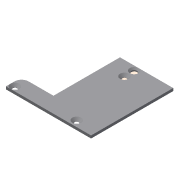
# Autodesk Inventor part: 11_Smartphone_Platform
Saved by Autodesk Inventor 2016 (Build 200138000, 138)
## iProperties
Created: 2017-01-03
Part Number: 11_Smartphone_Platform
Material: Generisch
Document SubType Name: Modeling
Designer: diederichbenedict
Density: 1 g/cm^3
Appearance: Vorgabe
Author: diederichbenedict
Autodesk Inventor part; units mm, degrees
ref_plane "YZ Plane" through (0, 0, 0) normal (1, 0, 0) x (0, 1, 0)
ref_plane "XZ Plane" through (0, 0, 0) normal (0, 1, 0) x (-1, 0, 0)
ref_plane "XY Plane" through (0, 0, 0) normal (0, 0, 1) x (1, 0, 0)
ref_plane "Arbeitsebene1" through (0, 0, 0) normal (0, 0, 1) x (1, 0, 0)
sketch "Skizze1" plane through (0, 0, 0) normal (0, 0, 1) x (1, 0, 0)
  circle A0 centre (-34, -41.2095) radius 2.25 projected
  line L0 (-29.75, -46.3143) -> (-39, -46.3143) projected
  line L1 (-29.75, -28.7171) -> (-29.75, -46.3143) projected
  line L2 (-31, -28.7171) -> (-29.75, -28.7171) projected
  arc A1 (-31, -28.7171) -> (-39, -36.7171) centre (-31, -36.7171) ccw projected
  line L3 (-39, -46.3143) -> (-39, -36.7171) projected
  line L4 (22, 46.3143) -> (22, 27.3143) projected
  line L5 (14, 46.3143) -> (22, 46.3143) projected
  line L6 (14, 27.3143) -> (14, 46.3143) projected
  line L7 (22, 27.3143) -> (14, 27.3143) projected
  circle A2 centre (18, 30.3143) radius 2.25 projected
  circle A3 centre (18, 41.3143) radius 3.2 projected
  line L8 (39, -36.6857) -> (39, -43.7095) projected
  arc A4 (39, -36.6857) -> (31, -28.6857) centre (31, -36.6857) ccw projected
  line L9 (30, -28.6857) -> (31, -28.6857) projected
  arc A5 (22, -20.6857) -> (30, -28.6857) centre (30, -20.6857) ccw projected
  line L10 (22, -18.1808) -> (22, -20.6857) projected
  line L11 (20, -18.1808) -> (22, -18.1808) projected
  line L12 (20, -43.7095) -> (20, -18.1808) projected
  line L13 (39, -43.7095) -> (20, -43.7095) projected
  circle A6 centre (34, -39.4595) radius 2.25 projected
  circle A7 centre (34, -58.6857) radius 4.25 construction
  circle A8 centre (-34, -58.6857) radius 4.25 construction
  circle A9 centre (18, 41.3143) radius 3.2 construction
  circle A10 centre (34, -39.4595) radius 2.25 construction
  circle A11 centre (-34, -41.2095) radius 2.25 construction
  circle A12 centre (18, 30.3143) radius 2.25 construction
  circle A13 centre (18, -14.7167) radius 2 construction
  circle A14 centre (18, 8.8143) radius 2 construction
  circle A15 centre (3.8024, -65.6857) radius 18.5 construction
  circle A16 centre (3, -8.6688) radius 3.05 construction
  arc A17 (-31, -28.7171) -> (-39, -36.7171) centre (-31, -36.7171) ccw construction
  line L14 (-11, -28.7171) -> (-31, -28.7171) construction
  arc A18 (-11, -28.7171) -> (-3, -20.7171) centre (-11, -20.7171) ccw construction
  line L15 (-3, 17.3143) -> (-3, -20.7171) construction
  arc A19 (5, 25.3143) -> (-3, 17.3143) centre (5, 17.3143) ccw construction
  line L16 (14, 25.3143) -> (5, 25.3143) construction
  line L17 (14, 46.3143) -> (14, 25.3143) construction
  line L18 (22, 46.3143) -> (14, 46.3143) construction
  line L19 (22, -20.6857) -> (22, 46.3143) construction
  arc A20 (22, -20.6857) -> (30, -28.6857) centre (30, -20.6857) ccw construction
  line L20 (31, -28.6857) -> (30, -28.6857) construction
  arc A21 (39, -36.6857) -> (31, -28.6857) centre (31, -36.6857) ccw construction
  line L21 (39, -79.0756) -> (39, -36.6857) construction
  arc A22 (31, -87.0756) -> (39, -79.0756) centre (31, -79.0756) ccw construction
  line L22 (-31, -87.0756) -> (31, -87.0756) construction
  arc A23 (-39, -79.0756) -> (-31, -87.0756) centre (-31, -79.0756) ccw construction
  line L23 (-39, -36.7171) -> (-39, -79.0756) construction
  circle A24 centre (3, 16.3312) radius 4 projected
  circle A25 centre (3, -33.6688) radius 4 projected
  circle A26 centre (3, 16.3312) radius 7.6 projected
  circle A27 centre (3, 16.3312) radius 4 projected
  circle A28 centre (3, 16.3312) radius 6 projected
  circle A29 centre (3, 16.3312) radius 6 projected
  line L24 (-39, -46.3143) -> (39, -46.3143)
  line L25 (39, -46.3143) -> (39, -43.7095)
  line L26 (-29.75, -28.7171) -> (-3, -28.7171)
  line L27 (-3, -28.7171) -> (-3, 46.3143)
  line L28 (-3, 46.3143) -> (22, 46.3143)
  line L29 (22, 46.3143) -> (22, -18.1808)
  line L30 (22, 46.3143) -> (57, 46.3143)
  line L31 (57, 46.3143) -> (57, -37.6857)
  line L32 (57, -37.6857) -> (22, -37.6857)
  line L33 (22, -37.6857) -> (22, 46.3143)
  line L34 (39, -46.3143) -> (57, -46.3143)
  line L35 (57, -46.3143) -> (57, -37.6857)
  line L36 (57, -37.6857) -> (39, -37.6857)
  line L37 (39, -37.6857) -> (39, -46.3143)
  point P0 (0, 0)
  dimension "d10" = 84
  dimension "d11" = 60
  constraints: 28 end point, 4 horizontal, 4 parallel, 3 perpendicular, 2 collinear, 2 point on line
  measures "d10" distance of L30.end L31.end
  measures "d11" distance between parallel lines of L31 L27
extrude "Extrusion1" add sketch "Skizze1" along normal blind 3 contours L0 L3 A1 L2 L1 | L1 L26 L27 A26 L28 L6 L7 L29 L11 L12 L13 L25 L24 | L25 L8 L32 L35 L34 | L13 L12 L11 L10 L33 L32 A6 L8 | A28 | L27 A26 | L32 A6 L33 A5 L9 A4 L8 | L8 A4 L9 A5 L10 L29 L4 L30 L31 L32 | L32 A6 | L4 L7 L6 L5 | A24 | A25 picked at (9.931, 15.2305) picked at (34.3207, -37.599)
sketch "Skizze2" plane through (0, 0, 0) normal (0, 0, -1) x (-1, 0, 0)
  circle A0 centre (-3, 16.3312) radius 4 projected
  circle A1 centre (-3, -33.6688) radius 4 projected
  circle A2 centre (-3, 16.3312) radius 4.3
  circle A3 centre (-3, -33.6688) radius 4.3
  circle A4 centre (-3, 16.3312) radius 6
  circle A5 centre (-3, -33.6688) radius 6
  point P0 (0, 0)
  dimension "d2" = 0.3
  dimension "d3" = 0.3
  dimension "d4" = 1.7
  dimension "d5" = 1.7
  constraints: 4 centre point
  measures "d2" radial gap between concentric circles of A0 A2
  measures "d3" radial gap between concentric circles of A1 A3
  measures "d4" radial gap between concentric circles of A2 A4
  measures "d5" radial gap between concentric circles of A3 A5
extrude "Extrusion2" add sketch "Skizze2" along normal blind 3 contours A4 | A5
sketch "Skizze3" plane through (0, 0, 3) normal (0, 0, 1) x (1, 0, 0)
  circle A0 centre (18, 41.3143) radius 3.2 projected
  circle A1 centre (18, 30.3143) radius 2.25 projected
  arc A2 (32.6157, -37.6857) -> (35.3843, -37.6857) centre (34, -39.4595) ccw projected
  circle A3 centre (-34, -41.2095) radius 2.25 projected
  point P0 (0, 0)
hole "Bohrung1" at (18, 41.3143, 3) at (18, 30.3143, 3) at (34, -39.4595, 3) at (-34, -41.2095, 3) direction (0, 0, -1) diameter 4 end through all countersink diameter 10 countersink angle 90
